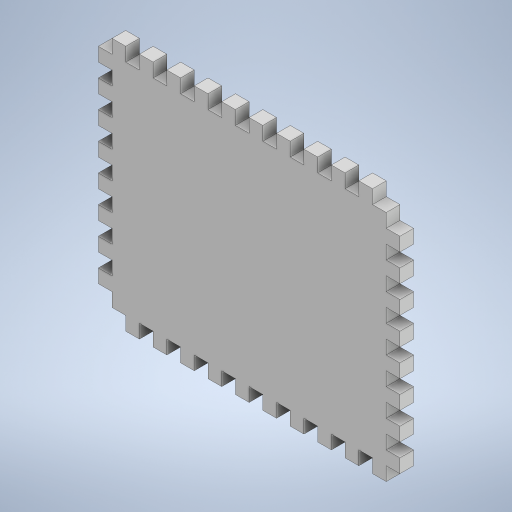
# Autodesk Inventor part: topside
Saved by Autodesk Inventor 2024 (Build 280153000, 153)
## iProperties
Created: 2024-04-15
Part Number: topside
Material: Generic
Document SubType Name: Modeling
Designer: srika
Density: 1 g/cm^3
Appearance: Default
Author: srika
Autodesk Inventor part; units mm, degrees
ref_plane "YZ Plane" through (0, 0, 0) normal (1, 0, 0) x (0, 1, 0)
ref_plane "XZ Plane" through (0, 0, 0) normal (0, 1, 0) x (-1, 0, 0)
ref_plane "XY Plane" through (0, 0, 0) normal (0, 0, 1) x (1, 0, 0)
sketch "Sketch1" plane through (0, 0, 0) normal (0, 0, 1) x (1, 0, 0)
  line L0 (5, 5) -> (105, 5)
  line L1 (105, 5) -> (105, 85)
  line L2 (105, 85) -> (5, 85)
  line L3 (5, 85) -> (5, 5)
  line L4 (0, 0) -> (5, 0)
  line L5 (5, 0) -> (5, 5)
  line L6 (5, 5) -> (0, 5)
  line L7 (0, 5) -> (0, 0)
  line L8 (0, 15) -> (0, 10)
  line L9 (5, 15) -> (0, 15)
  line L10 (0, 10) -> (5, 10)
  line L11 (0, 25) -> (0, 20)
  line L12 (5, 25) -> (0, 25)
  line L13 (0, 20) -> (5, 20)
  line L14 (0, 35) -> (0, 30)
  line L15 (5, 35) -> (0, 35)
  line L16 (0, 30) -> (5, 30)
  line L17 (0, 45) -> (0, 40)
  line L18 (5, 45) -> (0, 45)
  line L19 (0, 40) -> (5, 40)
  line L20 (0, 55) -> (0, 50)
  line L21 (5, 55) -> (0, 55)
  line L22 (0, 50) -> (5, 50)
  line L23 (0, 65) -> (0, 60)
  line L24 (5, 65) -> (0, 65)
  line L25 (0, 60) -> (5, 60)
  line L26 (0, 75) -> (0, 70)
  line L27 (5, 75) -> (0, 75)
  line L28 (0, 70) -> (5, 70)
  line L29 (0, 85) -> (0, 80)
  line L30 (5, 85) -> (0, 85)
  line L31 (0, 80) -> (5, 80)
  line L32 (10, 5) -> (10, 0)
  line L33 (10, 0) -> (15, 0)
  line L34 (15, 0) -> (15, 5)
  line L35 (20, 5) -> (20, 0)
  line L36 (20, 0) -> (25, 0)
  line L37 (25, 0) -> (25, 5)
  line L38 (30, 5) -> (30, 0)
  line L39 (30, 0) -> (35, 0)
  line L40 (35, 0) -> (35, 5)
  line L41 (40, 5) -> (40, 0)
  line L42 (40, 0) -> (45, 0)
  line L43 (45, 0) -> (45, 5)
  line L44 (50, 5) -> (50, 0)
  line L45 (50, 0) -> (55, 0)
  line L46 (55, 0) -> (55, 5)
  line L47 (60, 5) -> (60, 0)
  line L48 (60, 0) -> (65, 0)
  line L49 (65, 0) -> (65, 5)
  line L50 (70, 5) -> (70, 0)
  line L51 (70, 0) -> (75, 0)
  line L52 (75, 0) -> (75, 5)
  line L53 (80, 5) -> (80, 0)
  line L54 (80, 0) -> (85, 0)
  line L55 (85, 0) -> (85, 5)
  line L56 (90, 5) -> (90, 0)
  line L57 (90, 0) -> (95, 0)
  line L58 (95, 0) -> (95, 5)
  line L59 (100, 5) -> (100, 0)
  line L60 (100, 0) -> (105, 0)
  line L61 (105, 0) -> (105, 5)
  line L62 (105, 85) -> (110, 85)
  line L63 (110, 85) -> (110, 90)
  line L64 (110, 90) -> (105, 90)
  line L65 (105, 90) -> (105, 85)
  line L66 (105, 75) -> (110, 75)
  line L67 (110, 75) -> (110, 80)
  line L68 (110, 80) -> (105, 80)
  line L69 (105, 65) -> (110, 65)
  line L70 (110, 65) -> (110, 70)
  line L71 (110, 70) -> (105, 70)
  line L72 (105, 55) -> (110, 55)
  line L73 (110, 55) -> (110, 60)
  line L74 (110, 60) -> (105, 60)
  line L75 (105, 45) -> (110, 45)
  line L76 (110, 45) -> (110, 50)
  line L77 (110, 50) -> (105, 50)
  line L78 (105, 35) -> (110, 35)
  line L79 (110, 35) -> (110, 40)
  line L80 (110, 40) -> (105, 40)
  line L81 (105, 25) -> (110, 25)
  line L82 (110, 25) -> (110, 30)
  line L83 (110, 30) -> (105, 30)
  line L84 (105, 15) -> (110, 15)
  line L85 (110, 15) -> (110, 20)
  line L86 (110, 20) -> (105, 20)
  line L87 (105, 5) -> (110, 5)
  line L88 (110, 5) -> (110, 10)
  line L89 (110, 10) -> (105, 10)
  line L90 (100, 85) -> (100, 90)
  line L91 (100, 90) -> (95, 90)
  line L92 (95, 90) -> (95, 85)
  line L93 (90, 85) -> (90, 90)
  line L94 (90, 90) -> (85, 90)
  line L95 (85, 90) -> (85, 85)
  line L96 (80, 85) -> (80, 90)
  line L97 (80, 90) -> (75, 90)
  line L98 (75, 90) -> (75, 85)
  line L99 (70, 85) -> (70, 90)
  line L100 (70, 90) -> (65, 90)
  line L101 (65, 90) -> (65, 85)
  line L102 (60, 85) -> (60, 90)
  line L103 (60, 90) -> (55, 90)
  line L104 (55, 90) -> (55, 85)
  line L105 (50, 85) -> (50, 90)
  line L106 (50, 90) -> (45, 90)
  line L107 (45, 90) -> (45, 85)
  line L108 (40, 85) -> (40, 90)
  line L109 (40, 90) -> (35, 90)
  line L110 (35, 90) -> (35, 85)
  line L111 (30, 85) -> (30, 90)
  line L112 (30, 90) -> (25, 90)
  line L113 (25, 90) -> (25, 85)
  line L114 (20, 85) -> (20, 90)
  line L115 (20, 90) -> (15, 90)
  line L116 (15, 90) -> (15, 85)
  line L117 (10, 85) -> (10, 90)
  line L118 (10, 90) -> (5, 90)
  line L119 (5, 90) -> (5, 85)
  dimension "d0" = 100
  dimension "d1" = 80
  dimension "d4" = 10
  dimension "d11" = 10
  dimension "d16" = 5
  dimension "d17" = 5
  dimension "d20" = 10
  dimension "d27" = 10
  constraints: 236 end point, 80 horizontal alignment, 45 parallel, 20 collinear, 3 vertical, 2 horizontal, 2 perpendicular, 118 other
  measures "d0" distance of L3.start L1.end
  measures "d1" distance of L1.end L1.start
  measures "d4" distance of L4.start L8.end
  measures "d11" distance of L4.start L32.end
  measures "d16" distance of L64.end L63.end
  measures "d17" distance of L63.end L62.end
  measures "d20" distance of L62.end L66.end
  measures "d27" distance of L63.end L90.end
extrude "Extrusion1" add sketch "Sketch1" along normal blind 5 contours L3 L2 L1 L0 | L0 L34 L33 L32 | L10 L8 L9 L3 | L0 L37 L36 L35 | L13 L11 L12 L3 | L0 L40 L39 L38 | L16 L14 L15 L3 | L0 L43 L42 L41 | L19 L17 L18 L3 | L0 L46 L45 L44 | L22 L20 L21 L3 | L0 L49 L48 L47 | L25 L23 L24 L3 | L0 L52 L51 L50 | L28 L26 L27 L3 | L0 L55 L54 L53 | L31 L29 L30 L3 | L119 L118 L117 L2 | L0 L58 L57 L56 | L116 L115 L114 L2 | L0 L61 L60 L59 | L1 L89 L88 L87 | L113 L112 L111 L2 | L1 L86 L85 L84 | L110 L109 L108 L2 | L1 L83 L82 L81 | L107 L106 L105 L2 | L1 L80 L79 L78 | L104 L103 L102 L2 | L1 L77 L76 L75 | L101 L100 L99 L2 | L1 L74 L73 L72 | L98 L97 L96 L2 | L1 L71 L70 L69 | L95 L94 L93 L2 | L1 L68 L67 L66 | L92 L91 L90 L2
body "Solid1"
